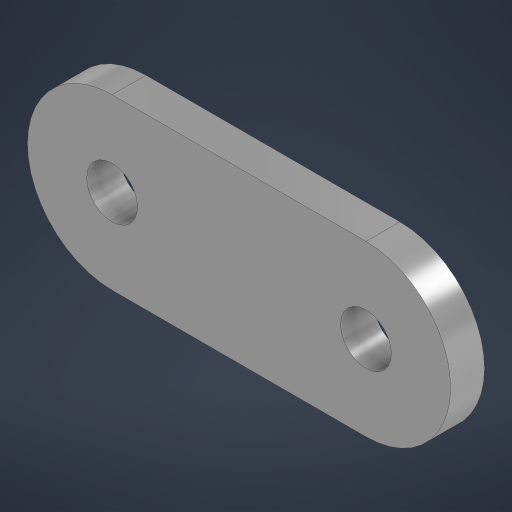
# Autodesk Inventor part: Middle support
Saved by Autodesk Inventor 2023 (Build 270158000, 158)
## iProperties
Created: 2023-04-12
Part Number: Middle support
Material: Generic
Document SubType Name: Modeling
Designer: vatdu
Density: 1 g/cm^3
Appearance: Default
Author: vatdu
Autodesk Inventor part; units mm, degrees
ref_plane "YZ Plane" through (0, 0, 0) normal (1, 0, 0) x (0, 1, 0)
ref_plane "XZ Plane" through (0, 0, 0) normal (0, 1, 0) x (-1, 0, 0)
ref_plane "XY Plane" through (0, 0, 0) normal (0, 0, 1) x (1, 0, 0)
sketch "Sketch1" plane through (0, 0, 0) normal (0, 0, 1) x (1, 0, 0)
  line L0 (0, 0) -> (25, 0)
  line L1 (25, 0) -> (25, 10)
  line L2 (25, 10) -> (0, 10)
  line L3 (0, 10) -> (0, 0)
  dimension "d0" = 25
  dimension "d1" = 10
  constraints: 8 end point, 2 parallel, 1 horizontal, 1 perpendicular
  measures "d0" distance of L2.end L1.end
  measures "d1" distance of L1.end L0.end
extrude "Extrusion1" add sketch "Sketch1" along normal blind 2
fillet "Fillet1" radius 5 4 edges at (25, 10, 1) (25, 0, 1) (0, 0, 1) (0, 10, 1)
sketch "Sketch2" plane through (0, 0, 2) normal (0, 0, 1) x (1, 0, 0)
  arc A0 (5, 10) -> (5, 0) centre (5, 5) ccw projected
  circle A1 centre (5, 5) radius 1.5
  arc A2 (20, 0) -> (20, 10) centre (20, 5) ccw projected
  circle A3 centre (20, 5) radius 1.5
  point P0 (0, 0)
  dimension "d5" = 3
  dimension "d6" = 3
  constraints: 2 centre point, 2 coincident
  measures "d5" diameter of A1
  measures "d6" diameter of A3
extrude "Extrusion2" cut sketch "Sketch2" against normal blind 2
body "Solid1"
